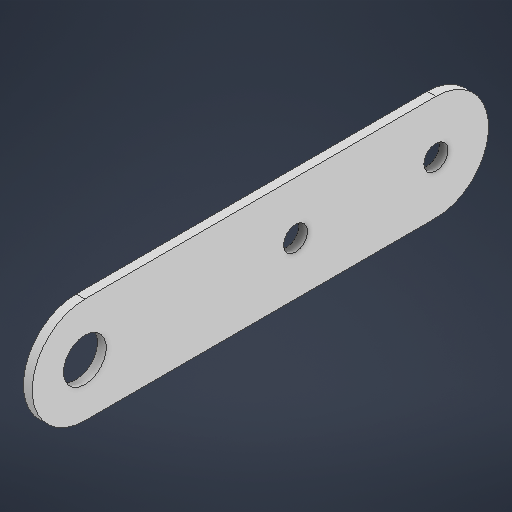
# Autodesk Inventor part: secondpreroller
Saved by Autodesk Inventor 2025.2 (Build 292293000, 293)
## iProperties
Created: 2025-04-08
Part Number: secondpreroller
Material: Generic
Document SubType Name: Modeling
Designer: roejo
Density: 1 g/cm^3
Appearance: Default
Author: roejo
Autodesk Inventor part; units mm, degrees
ref_plane "YZ Plane" through (0, 0, 0) normal (1, 0, 0) x (0, 1, 0)
ref_plane "XZ Plane" through (0, 0, 0) normal (0, 1, 0) x (-1, 0, 0)
ref_plane "XY Plane" through (0, 0, 0) normal (0, 0, 1) x (1, 0, 0)
sketch "Sketch1" plane through (0, 0, 0) normal (1, 0, 0) x (0, 1, 0)
  circle A0 centre (0, 0) radius 3.8735
  circle A1 centre (0, 0) radius 9.525
  circle A2 centre (0, -63.5) radius 2.1844
  circle A3 centre (0, -63.5) radius 9.525
  circle A4 centre (0, -38.1) radius 2.1844
  line L0 (9.525, 0) -> (9.525, -63.5)
  line L1 (-9.525, -63.5) -> (-9.525, 0)
  dimension "d0" = 7.747
  dimension "d1" = 19.05
  dimension "d2" = 4.3688
  dimension "d3" = 63.5
  dimension "d4" = 19.05
  dimension "d9" = 4.3688
  constraints: 5 centre point, 4 end point, 4 point on circle, 3 coincident, 1 parallel, 1 vertical
  measures "d0" diameter of A0
  measures "d1" diameter of A1
  measures "d2" diameter of A2
  measures "d3" distance of A2.centre point (0, 0)
  measures "d4" diameter of A3
  measures "d9" diameter of A4
extrude "Extrusion1" add sketch "Sketch1" along normal blind 1.5875
body "Solid1"
